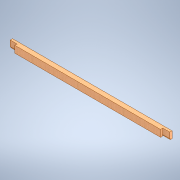
# Autodesk Inventor part: topv2
Saved by Autodesk Inventor 2020 (Build 240168000, 168)
## iProperties
Created: 2020-05-19
Part Number: topv2
Material: Wood (Cherry)
Document SubType Name: Modeling
Designer: kolbe
Density: 0.63 g/cm^3
Appearance: Cherry - Natural Low Gloss
Author: kolbe
Autodesk Inventor part; units mm, degrees
ref_plane "YZ Plane" through (0, 0, 0) normal (1, 0, 0) x (0, 1, 0)
ref_plane "XZ Plane" through (0, 0, 0) normal (0, 1, 0) x (-1, 0, 0)
ref_plane "XY Plane" through (0, 0, 0) normal (0, 0, 1) x (1, 0, 0)
sketch "Sketch1" plane through (0, 0, 0) normal (0, 0, 1) x (1, 0, 0)
  line L0 (0, 0) -> (889, 0)
  line L1 (889, 0) -> (889, 38.1)
  line L2 (889, 38.1) -> (0, 38.1)
  line L3 (0, 38.1) -> (0, 0)
  dimension "d0" = 889
  dimension "d1" = 38.1
  constraints: 8 end point, 2 parallel, 1 horizontal, 1 perpendicular
  measures "d0" distance of L2.end L1.end
  measures "d1" distance of L1.end L0.end
extrude "Extrusion1" add sketch "Sketch1" along normal blind 25.4
sketch "Sketch2" plane through (0, 0, 25.4) normal (0, 0, 1) x (1, 0, 0)
  line L0 (0, 38.1) -> (0, 0) projected
  line L1 (0, 0) -> (38.1, 0)
  line L2 (38.1, 0) -> (38.1, 38.1)
  line L3 (38.1, 38.1) -> (0, 38.1)
  line L4 (0, 38.1) -> (0, 0)
  line L5 (0, 0) -> (889, 0) projected
  line L6 (889, 0) -> (850.9, 0)
  line L7 (850.9, 0) -> (850.9, 38.1)
  line L8 (850.9, 38.1) -> (889, 38.1)
  line L9 (889, 38.1) -> (889, 0)
  dimension "d4" = 38.1
  dimension "d5" = 38.1
  dimension "d6" = 38.1
  dimension "d7" = 38.1
  constraints: 16 end point, 4 parallel, 2 horizontal, 2 perpendicular
  measures "d4" distance of L3.end L2.end
  measures "d5" distance of L2.end L1.end
  measures "d6" distance of L7.end L8.end
  measures "d7" distance of L6.end L7.end
extrude "Extrusion2" cut sketch "Sketch2" against normal blind 12.7 contours L7 L8 L9 L5
sketch "Sketch5" plane through (0, 0, 25.4) normal (0, 0, 1) x (1, 0, 0)
  line L0 (0, 0) -> (38.1, 0)
  line L1 (38.1, 0) -> (38.1, 38.1)
  line L2 (38.1, 38.1) -> (0, 38.1)
  line L3 (0, 38.1) -> (0, 0)
  dimension "d10" = 38.1
  dimension "d11" = 38.1
  constraints: 8 end point, 2 parallel, 1 horizontal, 1 perpendicular
  measures "d10" distance of L2.end L1.end
  measures "d11" distance of L1.end L0.end
extrude "Extrusion3" cut sketch "Sketch5" against normal blind 12.7
sketch "Sketch6" plane through (0, 0, 0) normal (0, -1, 0) x (1, 0, 0)
  line L0 (850.9, 12.7) -> (889, 12.7) projected
  line L1 (889, 12.7) -> (889, 9.525)
  line L2 (889, 0) -> (889, 12.7) projected
  line L3 (889, 9.525) -> (0, 9.525)
  line L4 (0, 9.525) -> (0, 15.875)
  line L5 (0, 15.875) -> (889, 15.875)
  line L6 (889, 15.875) -> (889, 12.7)
  dimension "d24" = 3.175
  dimension "d25" = 889
  dimension "d26" = 6.35
  dimension "d27" = 889
  constraints: 10 end point, 2 perpendicular, 2 point on line
  measures "d24" distance of L0.end L1.end
  measures "d25" distance of L1.end L3.end
  measures "d26" distance of L3.end L4.end
  measures "d27" distance of L4.end L5.end
extrude "Extrusion4" cut sketch "Sketch6" against normal blind 6.35
body "Solid1"
